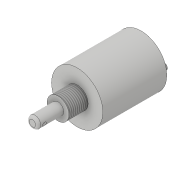
# Autodesk Inventor part: dc motor for capping system
Saved by Autodesk Inventor 2019 (Build 230136000, 136)
## iProperties
Created: 2019-10-12
Part Number: dc motor for capping system
Material: Generic
Document SubType Name: Modeling
Designer: Admin
Density: 1 g/cm^3
Appearance: Default
Author: Admin
Autodesk Inventor part; units mm, degrees
ref_plane "YZ Plane" through (0, 0, 0) normal (1, 0, 0) x (0, 1, 0)
ref_plane "XZ Plane" through (0, 0, 0) normal (0, 1, 0) x (-1, 0, 0)
ref_plane "XY Plane" through (0, 0, 0) normal (0, 0, 1) x (1, 0, 0)
sketch "Sketch1" plane through (0, 0, 0) normal (0, 0, 1) x (1, 0, 0)
  circle A0 centre (0, 0) radius 20
  dimension "d0" = 40
  constraints: 1 centre point, 1 coincident
  measures "d0" diameter of A0
extrude "Extrusion1" add sketch "Sketch1" along normal blind 50
sketch "Sketch2" plane through (0, 0, 50) normal (0, 0, 1) x (1, 0, 0)
  circle A0 centre (0, 0) radius 8.5
  dimension "d3" = 17
  constraints: 1 centre point, 1 coincident
  measures "d3" diameter of A0
extrude "Extrusion2" add sketch "Sketch2" along normal blind 15
thread "Thread1" size "M17x1.5" class "6g" standard "ANSI Metric M Profile" full length
sketch "Sketch3" plane through (0, 0, 65) normal (0, 0, 1) x (1, 0, 0)
  circle A0 centre (0, 0) radius 4.5
  dimension "d8" = 9
  constraints: 1 centre point, 1 coincident
  measures "d8" diameter of A0
extrude "Extrusion3" add sketch "Sketch3" along normal blind 20
sketch "Sketch4" plane through (0, 0, 0) normal (1, 0, 0) x (0, 1, 0)
  line L0 (4.5, 85) -> (-4.5, 85) projected
  line L1 (0, 85) -> (0, 80)
  circle A0 centre (0, 80) radius 1
  circle A1 centre (-1, 80) radius 1.5
  point P0 (0, 0)
  dimension "d11" = 5
  dimension "d12" = 3
  constraints: 2 end point, 1 centre point, 1 coincident, 1 horizontal alignment, 1 midpoint, 1 vertical, 2 other
  measures "d11" distance of L1.start L1.end
  measures "d12" diameter of A1
extrude "Extrusion4" cut sketch "Sketch4" along normal through all both and the other way through all contours A1 A0 L1 | L1 A0 A1 | A0 A1 picked at (0.0001, 79.7835)
fillet "Fillet1" radius 2 1 edges at (-4.5, 0, 85)
sketch "Sketch5" plane through (0, 0, 0) normal (0, 0, -1) x (-1, 0, 0)
  circle A0 centre (14, 0) radius 2.5
  circle A1 centre (-13, 0) radius 2.5
  point P0 (0, 0)
  dimension "d16" = 5
  dimension "d17" = 5
  constraints: 2 centre point
  measures "d16" diameter of A0
  measures "d17" diameter of A1
extrude "Extrusion5" add sketch "Sketch5" along normal blind 5
body "Solid1"
